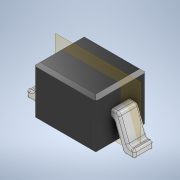
# Autodesk Inventor part: Part5
Saved by Autodesk Inventor 2021 (Build 250183000, 183)
## iProperties
Created: 2023-04-01
Part Number: Part5
Material: Generic
Document SubType Name: Modeling
Designer: stepa
Density: 1 g/cm^3
Appearance: Default
Author: stepa
Autodesk Inventor part; units mm, degrees
ref_plane "YZ Plane" through (0, 0, 0) normal (1, 0, 0) x (0, 1, 0)
ref_plane "XZ Plane" through (0, 0, 0) normal (0, 1, 0) x (-1, 0, 0)
ref_plane "XY Plane" through (0, 0, 0) normal (0, 0, 1) x (1, 0, 0)
sketch "Sketch1" plane through (0, 0, 0) normal (1, 0, 0) x (0, 1, 0)
  line L0 (0.65, 0.65) -> (-0.65, 0.65)
  line L1 (-0.65, 0.65) -> (-0.65, -0.65)
  line L2 (-0.65, -0.65) -> (0.65, -0.65)
  line L3 (0.65, -0.65) -> (0.65, 0.65)
  line L4 (0.65, 0.65) -> (-0.65, -0.65) construction
  line L5 (-0.65, 0.65) -> (0.65, -0.65) construction
  point P0 (0, 0)
  dimension "d0" = 1.3
  dimension "d1" = 1.3
  constraints: 12 end point, 2 midpoint, 2 parallel, 1 horizontal, 1 perpendicular
  measures "d0" distance of L2.end L1.end
  measures "d1" distance between parallel lines of L0 L2
extrude "Extrusion1" add sketch "Sketch1" along normal mid plane 1.6
chamfer "Chamfer1" distance 0.08 angle 45 8 edges at (0, 0.65, 0.65) (0, 0.65, -0.65) (0.8, 0.65, 0) (-0.8, 0.65, 0) (0, -0.65, 0.65) (0.8, -0.65, 0) (0, -0.65, -0.65) (-0.8, -0.65, 0)
ref_plane "Work Plane1" through (-0.8, -0.57, 0) normal (0, 0, 1) x (1, 0, 0)
sketch "Sketch2" plane through (-0.8, -0.57, 0) normal (0, 0, 1) x (1, 0, 0)
  line L0 (1.6, 0) -> (0, 0) projected
  line L1 (1.6, 1.14) -> (1.6, 0) projected
  line L2 (0, 1.14) -> (1.6, 1.14) projected
  line L3 (0, 0) -> (0, 1.14) projected
  line L4 (1.52, 1.22) -> (1.6, 1.14) projected
  line L5 (1.6, 1.14) -> (1.6, 0) projected
  line L6 (1.6, 0) -> (1.52, -0.08) projected
  line L7 (1.52, -0.08) -> (0.08, -0.08) projected
  line L8 (0.08, -0.08) -> (0, 0) projected
  line L9 (0, 0) -> (0, 1.14) projected
  line L10 (0, 1.14) -> (0.08, 1.22) projected
  line L11 (0.08, 1.22) -> (1.52, 1.22) projected
  line L12 (1.6, 1.14) -> (1.6, 0) projected
  line L13 (1.6, 0.57) -> (1.5908, 0.57)
  line L14 (1.6841, 0.5058) -> (1.8841, -0.0158)
  line L15 (1.9775, -0.08) -> (2.15, -0.08)
  line L16 (2.2, -0.03) -> (2.2, 0.07)
  line L17 (2.15, 0.12) -> (2.115, 0.12)
  line L18 (2.0216, 0.1842) -> (1.8217, 0.7058)
  line L19 (1.7283, 0.77) -> (1.6, 0.77)
  arc A0 (1.8217, 0.7058) -> (1.7283, 0.77) centre (1.7283, 0.67) ccw
  arc A1 (2.0216, 0.1842) -> (2.115, 0.12) centre (2.115, 0.22) ccw
  arc A2 (1.8841, -0.0158) -> (1.9775, -0.08) centre (1.9775, 0.02) ccw
  arc A3 (1.6841, 0.5058) -> (1.5908, 0.57) centre (1.5908, 0.47) ccw
  arc A4 (2.2, 0.07) -> (2.15, 0.12) centre (2.15, 0.07) ccw
  arc A5 (2.15, -0.08) -> (2.2, -0.03) centre (2.15, -0.03) ccw
  point P0 (0.8, 0.57)
  point P1 (1.6595, 0.57)
  point P2 (1.9087, -0.08)
  point P3 (2.2, -0.08)
  point P4 (2.2, 0.12)
  point P5 (2.0462, 0.12)
  point P6 (1.7971, 0.77)
  dimension "d7" = 0.2
  dimension "d8" = 0.2
  dimension "d9" = 0.2
  dimension "d10" = 0.6
  dimension "d11" = 0
  dimension "d14" = 0.1
  dimension "d15" = 0.05
  constraints: 14 end point, 13 point on line, 12 point on circle, 12 tangent, 6 centre point, 4 equal radius, 3 parallel, 2 perpendicular, 1 horizontal, 1 midpoint, 1 other
  measures "d7" distance between parallel lines of L13 L19
  measures "d8" distance between parallel lines of L18 L14
  measures "d9" distance between parallel lines of L17 L15
  measures "d10" distance between parallel lines of L1 L16
  measures "d11" distance between parallel lines of L15 L7
  measures "d14" radius of A0
  measures "d15" radius of A4
extrude "Extrusion2" add sketch "Sketch2" along normal mid plane 0.5 contours L1 L19 A0 L18 A1 L17 A4 L16 A5 L15 A2 L14 A3
fillet "Fillet1" radius 0.05 24 edges at (0.985, 0.1824, 0.25) (0.8641, 0.2, 0.25) (1.2583, -0.4324, 0.25) (1.3325, -0.45, 0.25) (1.3854, -0.4646, 0.25) (1.4, -0.55, 0.25) (1.3854, -0.6354, 0.25) (1.2637, -0.65, 0.25) (1.1208, -0.6324, 0.25) (0.9841, -0.325, 0.25) (0.8512, -0.0203, 0.25) (1.1216, -0.125, 0.25) (1.2583, -0.4324, -0.25) (1.3325, -0.45, -0.25) (1.3854, -0.4646, -0.25) (1.4, -0.55, -0.25) (1.3854, -0.6354, -0.25) (1.2637, -0.65, -0.25) (1.1208, -0.6324, -0.25) (0.9841, -0.325, -0.25) (0.8512, -0.0203, -0.25) (0.985, 0.1824, -0.25) (0.8641, 0.2, -0.25) (1.1216, -0.125, -0.25)
fillet "Fillet2" radius 0.05 4 edges at (0.8, 0, -0.65) (0.8, 0, 0.65) (-0.8, 0, -0.65) (-0.8, 0, 0.65)
mirror "Mirror1" about plane through (0, 0, 0) normal (1, 0, 0) of "Fillet1", "Extrusion2"
body "Solid1"
